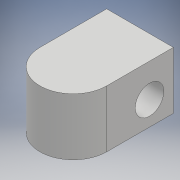
# Autodesk Inventor part: MissionTopEnd
Saved by Autodesk Inventor 2018.3 (Build 223284000, 284)
## iProperties
Created: 2018-07-21
Part Number: MissionTopEnd
Material: Generic
Document SubType Name: Modeling
Designer: mzhang
Density: 1 g/cm^3
Appearance: Default
Author: mzhang
Autodesk Inventor part; units mm, degrees
ref_plane "YZ Plane" through (0, 0, 0) normal (1, 0, 0) x (0, 1, 0)
ref_plane "XZ Plane" through (0, 0, 0) normal (0, 1, 0) x (-1, 0, 0)
ref_plane "XY Plane" through (0, 0, 0) normal (0, 0, 1) x (1, 0, 0)
sketch "Sketch1" plane through (0, 0, 0) normal (0, 0, 1) x (1, 0, 0)
  circle A0 centre (0, 0) radius 4
  arc A1 (-7, 0) -> (7, 0) centre (0, 0) ccw
  line L0 (-4, 0) -> (4, 0)
  line L1 (7, 0) -> (7, 14)
  line L2 (7, 14) -> (-7, 14)
  line L3 (-7, 14) -> (-7, 0)
  dimension "d0" = 8
  dimension "d1" = 3
  dimension "d2" = 14
  constraints: 8 end point, 4 point on circle, 2 centre point, 2 parallel, 1 coincident, 1 horizontal, 1 perpendicular
  measures "d0" diameter of A0
  measures "d1" radial gap between concentric circles of A0 A1
  measures "d2" distance of L1.end L1.start
extrude "Extrusion1" add sketch "Sketch1" along normal blind 10
sketch "Sketch2" plane through (7, 0, 0) normal (1, 0, 0) x (0, 0, -1)
  circle A0 centre (-5, 9) radius 3
  point P0 (0, 0)
  dimension "d5" = 6
  constraints: 1 centre point
  measures "d5" diameter of A0
extrude "Extrusion2" cut sketch "Sketch2" against normal blind 15
sketch "Sketch3" plane through (0, 0, 10) normal (0, 0, 1) x (1, 0, 0)
  circle A0 centre (0, 0) radius 4 projected
  arc A1 (-7, 0) -> (7, 0) centre (0, 0) ccw projected
  line L0 (7, 0) -> (7, 14) projected
  line L1 (7, 14) -> (-7, 14) projected
  line L2 (-7, 14) -> (-7, 0) projected
extrude "Extrusion3" add sketch "Sketch3" along normal blind 2 contours A0 | L2 L1 L0 A1
body "Solid1"
